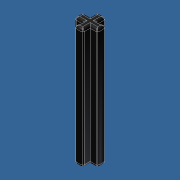
# Autodesk Inventor part: 4519
Saved by Autodesk Inventor 2011 SP2 (Build 150553200, 553)
## iProperties
Company: Allseas Engineering BV
Created: 2011-11-29
Part Number: 4519
Cost Center: 0 kg
Material: Steel
Document SubType Name: Modeling
Designer: PMe
Authority: 0 mm^3
Stock Number: =<Filenr>_<Document number>
Mass: 2.21403 g
Surface Area: 4.26022 cm^2
Volume: 0.282042 cm^3
Density: 7.85 g/cm^3
Act. Code: DW000
SaveDate: 2011-07-28
SaveTime: 18:32
FileName: Standard
TotalMass: 0 kg
TotalVolume: 0 mm^3
Subject: =<Title><TITLE 1_2> <TITLE 2_2>
Author: PMe
Autodesk Inventor part; units mm, degrees
ref_plane "YZ Plane" through (0, 0, 0) normal (1, 0, 0) x (0, 1, 0)
ref_plane "XZ Plane" through (0, 0, 0) normal (0, 1, 0) x (-1, 0, 0)
ref_plane "XY Plane" through (0, 0, 0) normal (0, 0, 1) x (1, 0, 0)
sketch "Sketch1" plane through (0, 0, 0) normal (0, 0, 1) x (1, 0, 0)
  circle A0 centre (0, 0) radius 2.3
  line L0 (-2.1564, 0.8) -> (-0.8, 0.8)
  line L1 (-0.8, 0.8) -> (-0.8, 2.1564)
  line L2 (0.8, 2.1564) -> (0.8, 0.8)
  line L3 (0.8, 0.8) -> (2.1564, 0.8)
  line L4 (2.1564, -0.8) -> (0.8, -0.8)
  line L5 (0.8, -0.8) -> (0.8, -2.1564)
  line L6 (-0.8, -2.1564) -> (-0.8, -0.8)
  line L7 (-0.8, -0.8) -> (-2.1564, -0.8)
  dimension "d0" = 4.6
  dimension "d1" = 1.6
  constraints: 16 end point, 4 perpendicular, 3 equal length, 3 parallel, 2 horizontal alignment, 2 vertical alignment, 1 coincident, 1 horizontal, 10 other
  measures "d1" distance between parallel lines of L2 L1
extrude "Extrusion1" add sketch "Sketch1" along normal mid plane 24 contours A0 L4 L5 L6 L7 L0 L1 L2 L3
fillet "Fillet1" radius 0.5 24 edges at (0, 2.3, 12) (0.8, 1.4782, 12) (1.4782, 0.8, 12) (2.3, 0, 12) (1.4782, -0.8, 12) (0.8, -1.4782, 12) (0, -2.3, 12) (-0.8, -1.4782, 12) (-1.4782, -0.8, 12) (-2.3, 0, 12) (-1.4782, 0.8, 12) (-0.8, 1.4782, 12) (0, 2.3, -12) (-2.3, 0, -12) (0, -2.3, -12) (2.3, 0, -12) (1.4782, 0.8, -12) (0.8, 1.4782, -12) (-0.8, 1.4782, -12) (-1.4782, 0.8, -12) (-1.4782, -0.8, -12) (-0.8, -1.4782, -12) (0.8, -1.4782, -12) (1.4782, -0.8, -12)
fillet "Fillet2" radius 0.2 24 edges at (0.8, 2.1564, 0) (0.6467, 2.047, 11.8603) (0.6467, 2.047, -11.8603) (-0.8, 2.1564, 0) (-0.6467, 2.047, 11.8603) (-0.6467, 2.047, -11.8603) (-2.1564, 0.8, 0) (-2.047, 0.6467, -11.8603) (-2.047, 0.6467, 11.8603) (-2.1564, -0.8, 0) (-2.047, -0.6467, 11.8603) (-2.047, -0.6467, -11.8603) (-0.8, -2.1564, 0) (-0.6467, -2.047, 11.8603) (-0.6467, -2.047, -11.8603) (0.8, -2.1564, 0) (0.6467, -2.047, 11.8603) (0.6467, -2.047, -11.8603) (2.1564, -0.8, 0) (2.047, -0.6467, 11.8603) (2.047, -0.6467, -11.8603) (2.1564, 0.8, 0) (2.047, 0.6467, 11.8603) (2.047, 0.6467, -11.8603)
body "Solid1"
